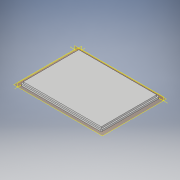
# Autodesk Inventor part: receiver-box-lid
Saved by Autodesk Inventor 2017 (Build 210142000, 142)
## iProperties
Created: 2020-06-15
Part Number: receiver-box-lid
Material: Generic
Document SubType Name: Modeling
Designer: HAYNIE R&D
Density: 1 g/cm^3
Appearance: Default
Author: HAYNIE R&D
Autodesk Inventor part; units mm, degrees
sketch "Sketch2" plane through (0, 0, 0) normal (0, 1, 0) x (-1, 0, 0)
  line L0 (8.6373, 10.8766) -> (-116.3627, 10.8766)
  line L1 (-116.3627, 10.8766) -> (-116.3627, -79.1234)
  line L2 (-116.3627, -79.1234) -> (8.6373, -79.1234)
  line L3 (8.6373, -79.1234) -> (8.6373, 10.8766)
  point P0 (0, 0)
  dimension "d1" = 125
  dimension "d2" = 90
  constraints: 8 end point, 2 parallel, 1 horizontal, 1 perpendicular
  measures "d1" distance of L2.end L1.end
  measures "d2" distance of L1.end L0.end
extrude "Extrusion1" add sketch "Sketch2" along normal blind 2.5
sketch "Sketch3" plane through (0, 2.5, 0) normal (0, 1, 0) x (1, 0, 0)
  line L0 (-6.3307, 76.9149) -> (114.3414, 76.9149)
  line L1 (114.3414, 76.9149) -> (114.3414, -8.9534)
  line L2 (114.3414, -8.9534) -> (-6.3307, -8.9534)
  line L3 (-6.3307, -8.9534) -> (-6.3307, 76.9149)
  point P0 (0, 0)
  constraints: 8 end point, 2 parallel, 1 horizontal, 1 perpendicular
extrude "Extrusion2" add sketch "Sketch3" along normal blind 2.5
fillet "Fillet1" radius 2 1 edges at (-8.6373, 1.25, 10.8766)
fillet "Fillet2" radius 2 1 edges at (116.3627, 1.25, 10.8766)
fillet "Fillet3" radius 2 1 edges at (116.3627, 1.25, -79.1234)
fillet "Fillet4" radius 2 1 edges at (-8.6373, 1.25, -79.1234)
move or copy body "Move Body1" bodies to move or copy 1 copy no translate (8.63, 0, 0)
move or copy body "Move Body2" bodies to move or copy 1 copy no translate (0, 0, 79.1)
body "Solid1"
